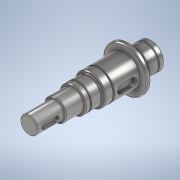
# Autodesk Inventor part: AbtriebswelleZahnrad 2
Saved by Autodesk Inventor 2022 (Build 260153000, 153)
## iProperties
Created: 2023-01-25
Part Number: AbtriebswelleZahnrad 2
Material: Stahl, Legierung
Document SubType Name: Modeling
Designer: Matias Nicky
Density: 7.73 g/cm^3
Appearance: Halbpoliert
Author: Matias Nicky
Autodesk Inventor part; units mm, degrees
ref_plane "XZ Plane" through (0, 0, 0) normal (0, 1, 0) x (-1, 0, 0)
sketch "Skizze1" plane through (0, 0, 0) normal (1, 0, 0) x (0, 1, 0)
  line L0 (0, 95) -> (10, 95)
  line L1 (10, 95) -> (10, 65)
  line L2 (10, 65) -> (12.5, 65)
  line L3 (12.5, 65) -> (12.5, 45)
  line L4 (12.5, 45) -> (15, 45)
  line L5 (17.5, -14.649) -> (25, -14.649)
  line L6 (25, -14.649) -> (25, -19.649)
  line L7 (25, -19.649) -> (17.5, -19.649)
  line L8 (17.5, -19.649) -> (17.5, -25)
  line L9 (15, -45) -> (0, -45)
  line L10 (0, 123) -> (0, -73) projected
  line L11 (-5, 0) -> (30, 0) projected
  line L12 (15, 45) -> (15, 39.6)
  line L13 (15, 39.6) -> (13.6, 39.6)
  line L14 (13.6, 39.6) -> (13.6, 38)
  line L15 (13.6, 38) -> (15, 38)
  line L16 (15, 38) -> (15, 27.5)
  line L17 (15, 27.5) -> (14.7, 26.3804)
  arc A0 (14.7, 26.3804) -> (14.6659, 26.1216) centre (15.6659, 26.1216) ccw
  arc A1 (14.6659, 25.8728) -> (15.7, 25) centre (15.6579, 25.9991) ccw
  line L18 (14.6659, 25.8728) -> (14.6659, 26.1216)
  line L19 (17.5, 25) -> (15.7, 25)
  line L20 (15, -45) -> (15, -39.6)
  line L21 (15, -39.6) -> (13.6, -39.6)
  line L22 (13.6, -39.6) -> (13.6, -38)
  line L23 (13.6, -38) -> (15, -38)
  line L24 (15, -38) -> (15, -27.5)
  line L25 (15, -27.5) -> (14.7341, -26.5076)
  line L26 (17.5, -25) -> (16, -25)
  line L27 (16, -25) -> (15.7, -25)
  arc A2 (15.7, -25) -> (14.7, -26) centre (15.7, -26) ccw
  arc A3 (14.7, -26.2487) -> (14.7341, -26.5076) centre (15.7, -26.2487) ccw
  line L28 (14.7, -26.2487) -> (14.7, -26)
  line L29 (17.5, 25) -> (17.5, 16.249)
  line L30 (17.5, 16.249) -> (15.5, 16.249)
  line L31 (15.5, 16.249) -> (15.5, 14.649)
  line L32 (15.5, 14.649) -> (17.5, 14.649)
  line L33 (17.5, 14.649) -> (17.5, -14.649)
  point P0 (0, 0)
  point P1 (14.6579, 24.9991)
  point P2 (14.7, -26.3804)
  point P3 (14.7, -25)
  dimension "d0" = 20
  dimension "d3" = 25
  dimension "d5" = 50
  dimension "d6" = 20
  dimension "d7" = 30
  dimension "d10" = 5
  dimension "d11" = 50
  dimension "d13" = 2.5
  dimension "d17" = 1
  dimension "d18" = 1
  dimension "d20" = 30
  dimension "d21" = 20
  dimension "d22" = 0.3
  dimension "d23" = 15
  dimension "d25" = 1.6
  dimension "d26" = 1.4
  dimension "d28" = 2.5
  dimension "d31" = 1
  dimension "d32" = 15
  dimension "d33" = 0.3
  dimension "d34" = 1
  dimension "d35" = 1.4
  dimension "d36" = 1.6
  dimension "d37" = 13
  dimension "d38" = 20
  dimension "d39" = 1.6
  dimension "d40" = 2
  dimension "d83" = 14.649
  dimension "d84" = 29.298
  dimension "d85" = 13
  dimension "d86" = 35
  constraints: 64 end point, 15 perpendicular, 9 point on line, 8 point on circle, 4 centre point, 4 tangent, 4 vertical, 2 horizontal, 1 equal radius, 1 symmetric about line
  measures "d0" diameter of L1 L10
  measures "d3" diameter of L3 L10
  measures "d5" distance of L8.end L19.start
  measures "d6" distance of L3.end L2.end
  measures "d7" distance of L1.end L0.end
  measures "d10" distance between parallel lines of L7 L5
  measures "d11" diameter of L6 L10
  measures "d13" horizontal distance of L19.start L16.end
  measures "d17" radius of A0
  measures "d18" horizontal distance of A1.centre point (14.658, 24.999)
  measures "d20" diameter of L4.end L10
  measures "d21" vertical distance of L19.start L4.end
  measures "d22" distance from line of L17.end L16
  measures "d23" angle of L18 L17
  measures "d25" distance of L15.end L12.end
  measures "d26" distance of L13.end L12.end
  measures "d28" horizontal distance of L8.end L24.end
  measures "d31" radius of A2
  measures "d32" angle of L24 L25
  measures "d33" distance from line of L24 point (14.7, -26.38)
  measures "d34" radius of A3
  measures "d35" distance between parallel lines of L22 L24
  measures "d36" distance between parallel lines of L21 L23
  measures "d37" distance from line of L8.end L23
  measures "d38" vertical distance of L8.end L9.start
  measures "d39" distance between parallel lines of L32 L30
  measures "d40" distance between parallel lines of L31 L29
  measures "d83" distance between parallel lines of L11 L5
  measures "d84" vertical distance of L5.end L32.end
  measures "d85" distance from line of L15 L19.start
  measures "d86" diameter of L8 L10
revolve "Umdrehung1" add sketch "Skizze1" angle 360 about axis through (0, 0, 0) along (0, 0, -1)
chamfer "Fase1" distance 1 angle 45 1 edges at (0, -10, 95) measured on face at (2.9244, -0.4018, 95)
chamfer "Fase2" distance 1 angle 45 1 edges at (0, -12.5, 65) measured on face at (-1.7949, 11.4487, 65)
chamfer "Fase3" distance 1 angle 45 1 edges at (0, -15, 45) measured on face at (-1.1966, 14.0214, 45)
chamfer "Fase4" distance 1 angle 45 1 edges at (0, -17.5, 25) measured on face at (-1.396, 16.7305, 25)
chamfer "Fase5" distance 1 angle 45 1 edges at (0, -25, -14.649) measured on face at (-1.9943, 22.2578, -14.649)
chamfer "Fase6" distance 1 angle 45 1 edges at (0, -25, -19.649) measured on face at (-3.3903, 22.0883, -19.649)
chamfer "Fase7" distance 1 angle 45 1 edges at (0, -17.5, -25) measured on face at (-1.396, 16.8305, -25)
chamfer "Fase8" distance 1 angle 45 1 edges at (0, -15, -45) measured on face at (2.9183, -2.695, -45)
ref_plane "Arbeitsebene1" through (10, 0, 0) normal (1, 0, 0) x (0, 1, 0)
sketch "Skizze2" plane through (10, 0, 0) normal (1, 0, 0) x (0, 1, 0)
  line L0 (0, 87) -> (0, 73) construction
  line L1 (-3, 87) -> (-3, 73)
  line L2 (3, 73) -> (3, 87)
  arc A0 (3, 87) -> (-3, 87) centre (0, 87) ccw
  arc A1 (-3, 73) -> (3, 73) centre (0, 73) ccw
  line L3 (-9, 95) -> (9, 95) projected
  point P0 (0, 0)
  point P1 (0, 80)
  dimension "d68" = 20
  dimension "d69" = 15
  dimension "d70" = 6
  constraints: 8 end point, 4 point on circle, 4 tangent, 2 centre point, 1 midpoint, 1 parallel, 1 vertical
  measures "d69" distance from line of L3 point (0, 80)
  measures "d70" distance between parallel lines of L1 L2
extrude "Extrusion1" cut sketch "Skizze2" against normal blind 3.55
ref_plane "Arbeitsebene2" through (17.5, 0, 0) normal (1, 0, 0) x (0, 1, 0)
sketch "Skizze3" plane through (17.5, 0, 0) normal (1, 0, 0) x (0, 1, 0)
  line L0 (0, 6) -> (0, -6) construction
  line L1 (-5, 6) -> (-5, -6)
  line L2 (5, -6) -> (5, 6)
  arc A0 (5, 6) -> (-5, 6) centre (0, 6) ccw
  arc A1 (-5, -6) -> (5, -6) centre (0, -6) ccw
  line L3 (-7, 0) -> (7, 0) projected
  point P0 (0, 0)
  point P1 (0, 0)
  dimension "d74" = 22
  dimension "d75" = 10
  constraints: 8 end point, 4 point on circle, 4 tangent, 2 centre point, 1 midpoint, 1 parallel, 1 symmetric about line, 1 vertical
  measures "d75" distance between parallel lines of L1 L2
extrude "Extrusion2" cut sketch "Skizze3" against normal blind 5 and the other way blind 1.45
equation "\"dd0\" = 6"
equation "\"dd1\" = 4"
